Autodesk Fusion 360 part; units mm, degrees
(part 19 of 25)
  line L2175 (67.3326, 33.4819) -> (67.1928, 33.6743)
  arc A5897 (67.71, 32.8087) -> (67.3925, 32.8087) centre (67.5513, 32.8087) ccw
  line L2176 (64.5, 34.1863) -> (63.8511, 34.4551)
  line L2177 (67.5513, 32.8087) -> (67.5141, 33.0437)
  line L2178 (66.1589, 34.2011) -> (66.04, 34.2011)
  line L2179 (59.1947, 30.4591) -> (59.4635, 29.8102)
  line L2180 (67.5513, 30.6913) -> (67.5513, 31.75)
  arc A5898 (59.8478, 29.2014) -> (60.0723, 29.4259) centre (59.9601, 29.3137) ccw
  line L2181 (63.1489, 34.4551) -> (62.5, 34.1863)
  arc A5899 (67.3212, 33.7677) -> (67.0643, 33.581) centre (67.1928, 33.6743) ccw
  arc A5900 (60.0208, 29.4603) -> (59.8993, 29.167) centre (59.9601, 29.3137) ccw
  line L2182 (59.96, 29.3137) -> (60.6089, 29.0449)
  arc A5901 (62.1177, 33.8041) -> (62.3423, 34.0286) centre (62.23, 33.9163) ccw
  arc A5902 (63.2096, 34.3084) -> (63.0881, 34.6018) centre (63.1489, 34.4551) ccw
  arc A5903 (61.8992, 34.0397) -> (62.0207, 34.333) centre (61.9599, 34.1864) ccw
  line L2183 (63.8511, 34.4551) -> (63.1489, 34.4551)
  arc A5904 (65.9211, 34.3598) -> (65.9211, 34.0423) centre (65.9211, 34.2011) ccw
  arc A5905 (64.8373, 33.6244) -> (65.0619, 33.849) centre (64.9496, 33.7367) ccw
  arc A5906 (65.3412, 33.8539) -> (65.1546, 34.1108) centre (65.2479, 33.9824) ccw
  arc A5907 (61.3719, 34.6018) -> (61.2504, 34.3084) centre (61.3112, 34.4551) ccw
  arc A5908 (62.1177, 34.0286) -> (62.3423, 33.8041) centre (62.23, 33.9164) ccw
  arc A5909 (59.3414, 30.5198) -> (59.048, 30.3983) centre (59.1947, 30.4591) ccw
  arc A5910 (66.04, 34.0423) -> (66.04, 34.3598) centre (66.04, 34.2011) ccw
  arc A5911 (62.0722, 34.2986) -> (61.8477, 34.0741) centre (61.9599, 34.1864) ccw
  arc A5912 (62.4393, 34.333) -> (62.5608, 34.0397) centre (62.5001, 34.1864) ccw
  line L2184 (59.1947, 33.0409) -> (59.1947, 30.4591)
  line L2185 (59.96, 34.1863) -> (59.4635, 33.6898)
  line L2186 (65.0555, 33.8426) -> (64.9496, 33.7367)
  line L2187 (65.9211, 34.2011) -> (65.6861, 34.1639)
  arc A5913 (63.8511, 34.2963) -> (63.8511, 34.6138) centre (63.8511, 34.455) ccw
  arc A5914 (65.7352, 34.0129) -> (65.637, 34.3149) centre (65.6861, 34.1639) ccw
  arc A5915 (63.1489, 34.6138) -> (63.1489, 34.2963) centre (63.1489, 34.455) ccw
  line L2188 (59.4635, 33.6898) -> (59.1947, 33.0409)
  arc A5916 (64.8373, 33.849) -> (65.0619, 33.6244) centre (64.9496, 33.7367) ccw
  arc A5917 (65.1758, 34.1238) -> (65.32, 33.8409) centre (65.2479, 33.9824) ccw
  arc A5918 (59.6101, 33.629) -> (59.3168, 33.7505) centre (59.4635, 33.6897) ccw
  arc A5919 (60.5481, 28.8982) -> (60.6696, 29.1916) centre (60.6089, 29.0449) ccw
  arc A5920 (60.6696, 34.3084) -> (60.5481, 34.6018) centre (60.6089, 34.4551) ccw
  arc A5921 (65.4108, 34.2414) -> (65.5089, 33.9394) centre (65.4599, 34.0904) ccw
  arc A5922 (60.0723, 34.0741) -> (59.8478, 34.2986) centre (59.9601, 34.1864) ccw
  line L2189 (65.4599, 34.0904) -> (65.2479, 33.9824)
  arc A5923 (59.3168, 29.7495) -> (59.6101, 29.871) centre (59.4635, 29.8102) ccw
  line L2190 (60.6089, 34.4551) -> (59.96, 34.1863)
  arc A5924 (59.3535, 33.0409) -> (59.036, 33.0409) centre (59.1947, 33.0409) ccw
  arc A5925 (61.3111, 28.8862) -> (61.3111, 29.2037) centre (61.3111, 29.045) ccw
  arc A5926 (62.6123, 34.0741) -> (62.3878, 34.2986) centre (62.5001, 34.1863) ccw
  line L2191 (59.4635, 29.8102) -> (59.96, 29.3137)
  arc A5927 (60.6089, 34.6138) -> (60.6089, 34.2963) centre (60.6089, 34.455) ccw
  arc A5928 (59.5757, 29.9225) -> (59.3512, 29.698) centre (59.4635, 29.8102) ccw
  arc A5929 (64.9621, 33.971) -> (65.1488, 33.7141) centre (65.0555, 33.8426) ccw
  line L2192 (65.6861, 34.1639) -> (65.4599, 34.0904)
  arc A5930 (61.3111, 34.2963) -> (61.3111, 34.6138) centre (61.3111, 34.455) ccw
  line L2193 (62.5, 34.1863) -> (62.23, 33.9163)
  line L2194 (61.3111, 34.4551) -> (60.6089, 34.4551)
  line L2195 (61.96, 34.1863) -> (61.3111, 34.4551)
  arc A5931 (65.5319, 33.9489) -> (65.3878, 34.2318) centre (65.4599, 34.0904) ccw
  arc A5932 (63.9119, 34.6018) -> (63.7904, 34.3084) centre (63.8512, 34.4551) ccw
  line L2196 (62.23, 33.9163) -> (61.96, 34.1863)
  line L2197 (65.2479, 33.9824) -> (65.0555, 33.8426)
  arc A5933 (59.3512, 33.802) -> (59.5757, 33.5775) centre (59.4635, 33.6898) ccw
  arc A5934 (65.1677, 33.7303) -> (64.9432, 33.9548) centre (65.0555, 33.8425) ccw
  arc A5935 (68.4212, 25.4) -> (68.7387, 25.4) centre (68.5799, 25.4) ccw
  line L2198 (67.3481, 25.4) -> (67.3481, 24.8897)
  arc A5936 (62.6433, 28.6748) -> (62.4188, 28.4503) centre (62.5311, 28.5626) ccw
  arc A5937 (69.342, 26.6382) -> (69.342, 26.9558) centre (69.342, 26.797) ccw
  line L2199 (68.58, 25.4) -> (67.3481, 25.4)
  arc A5938 (68.58, 25.5588) -> (68.58, 25.2413) centre (68.58, 25.4001) ccw
  line L2200 (68.58, 26.6319) -> (68.58, 25.4)
  arc A5939 (67.2358, 26.0225) -> (67.4604, 25.798) centre (67.3481, 25.9103) ccw
  line L2201 (67.3481, 25.4) -> (68.58, 25.4)
  arc A5940 (67.1894, 24.8897) -> (67.5069, 24.8897) centre (67.3482, 24.8897) ccw
  arc A5941 (61.2504, 29.1916) -> (61.3719, 28.8982) centre (61.3112, 29.0449) ccw
  arc A5942 (64.4819, 26.6503) -> (64.6034, 26.9437) centre (64.5426, 26.797) ccw
  arc A5943 (61.8477, 29.4259) -> (62.0722, 29.2014) centre (61.9599, 29.3137) ccw
  line L2202 (64.1225, 26.971) -> (64.5426, 26.797)
  arc A5944 (68.4213, 25.4) -> (68.7388, 25.4) centre (68.58, 25.4) ccw
  arc A5945 (62.2447, 29.3444) -> (62.4693, 29.5689) centre (62.357, 29.4567) ccw
  arc A5946 (62.3843, 28.5018) -> (62.6777, 28.6233) centre (62.531, 28.5626) ccw
  line L2203 (62.531, 28.5625) -> (63.801, 27.2925)
  arc A5947 (69.1833, 26.3802) -> (69.5007, 26.3802) centre (69.342, 26.3802) ccw
  line L2204 (64.5426, 26.797) -> (69.342, 26.797)
  arc A5948 (62.1983, 28.9826) -> (62.5158, 28.9826) centre (62.3571, 28.9826) ccw
  arc A5949 (68.58, 26.7906) -> (68.58, 26.4731) centre (68.58, 26.6319) ccw
  arc A5950 (63.9133, 27.4048) -> (63.6888, 27.1803) centre (63.801, 27.2926) ccw
  arc A5951 (67.5069, 25.9103) -> (67.1894, 25.9103) centre (67.3482, 25.9103) ccw
  arc A5952 (62.3423, 29.4714) -> (62.1177, 29.6959) centre (62.23, 29.5836) ccw
  arc A5953 (62.5158, 29.4567) -> (62.1983, 29.4567) centre (62.3571, 29.4567) ccw
  arc A5954 (69.0903, 26.4731) -> (69.0903, 26.7906) centre (69.0903, 26.6319) ccw
  arc A5955 (59.036, 30.4591) -> (59.3535, 30.4591) centre (59.1947, 30.4591) ccw
  arc A5956 (69.5007, 26.797) -> (69.1833, 26.797) centre (69.342, 26.797) ccw
  line L2205 (63.801, 27.2925) -> (64.1225, 26.971)
  arc A5957 (62.0207, 29.167) -> (61.8992, 29.4603) centre (61.9599, 29.3137) ccw
  line L2206 (62.357, 28.9826) -> (62.531, 28.5625)
  arc A5958 (68.4212, 25.4) -> (68.7387, 25.4) centre (68.5799, 25.4) ccw
  line L2207 (68.58, 26.6319) -> (68.0697, 26.6319)
  arc A5959 (64.0103, 26.8588) -> (64.2348, 27.0833) centre (64.1226, 26.9711) ccw
  arc A5960 (68.7387, 25.4) -> (68.4212, 25.4) centre (68.5799, 25.4) ccw
  line L2208 (64.9496, 33.7367) -> (64.5, 34.1863)
  arc A5961 (68.0697, 26.7906) -> (68.0697, 26.4731) centre (68.0697, 26.6319) ccw
  arc A5962 (64.6122, 34.2986) -> (64.3877, 34.0741) centre (64.5, 34.1864) ccw
  arc A5963 (67.3481, 25.5588) -> (67.3481, 25.2413) centre (67.3481, 25.4001) ccw
  line L2209 (62.23, 29.5837) -> (62.357, 29.4567)
  arc A5964 (68.58, 25.2413) -> (68.58, 25.5588) centre (68.58, 25.4001) ccw
  arc A5965 (67.3481, 25.5587) -> (67.3481, 25.2412) centre (67.3481, 25.4) ccw
  arc A5966 (68.58, 25.2413) -> (68.58, 25.5588) centre (68.58, 25.4001) ccw
  line L2210 (69.342, 26.797) -> (69.342, 26.3802)
  arc A5967 (68.58, 25.2412) -> (68.58, 25.5587) centre (68.58, 25.4) ccw
  arc A5968 (68.7387, 26.6319) -> (68.4212, 26.6319) centre (68.5799, 26.6319) ccw
  arc A5969 (62.5037, 29.0434) -> (62.2103, 28.9219) centre (62.357, 28.9827) ccw
  line L2211 (62.357, 29.4567) -> (62.357, 28.9826)
  arc A5970 (69.2297, 26.2679) -> (69.4543, 26.4924) centre (69.342, 26.3801) ccw
  arc A5971 (68.0697, 24.3268) -> (68.0697, 24.0094) centre (68.0697, 24.1681) ccw
  arc A5972 (68.58, 26.4731) -> (68.58, 26.7906) centre (68.58, 26.6319) ccw
  line L2212 (67.437, 18.8226) -> (67.611, 18.4025)
  arc A5973 (68.0768, 21.6936) -> (67.8523, 21.9182) centre (67.9646, 21.8059) ccw
  line L2213 (67.611, 18.4025) -> (67.9325, 18.081)
  line L2214 (68.58, 24.1681) -> (68.58, 25.4)
  arc A5974 (68.182, 26.5196) -> (67.9575, 26.7442) centre (68.0697, 26.6319) ccw
  arc A5975 (68.58, 25.2412) -> (68.58, 25.5587) centre (68.58, 25.4) ccw
  line L2215 (69.0903, 26.6319) -> (68.58, 26.6319)
  line L2216 (68.58, 25.4) -> (68.58, 26.6319)
  line L2217 (69.342, 26.3802) -> (69.0903, 26.6319)
  arc A5976 (72.9775, 15.7587) -> (72.753, 15.5341) centre (72.8653, 15.6464) ccw
  line L2218 (68.58, 25.4) -> (68.58, 24.1681)
  line L2219 (67.0941, 20.9355) -> (67.0941, 19.7045)
  arc A5977 (67.7233, 18.5148) -> (67.4988, 18.2903) centre (67.6111, 18.4026) ccw
  arc A5978 (69.4543, 22.5862) -> (69.2297, 22.8107) centre (69.342, 22.6985) ccw
  arc A5979 (64.5426, 26.9558) -> (64.5426, 26.6382) centre (64.5426, 26.797) ccw
  arc A5980 (68.7387, 25.4) -> (68.4212, 25.4) centre (68.5799, 25.4) ccw
  arc A5981 (70.2539, 15.9671) -> (70.1324, 15.6737) centre (70.1932, 15.8204) ccw
  line L2220 (72.8653, 15.6464) -> (73.2188, 15.2929)
  arc A5982 (69.2025, 26.7441) -> (68.978, 26.5196) centre (69.0902, 26.6319) ccw
  line L2221 (67.3481, 25.9103) -> (67.3481, 25.4)
  line L2222 (73.8677, 15.0241) -> (74.5699, 15.0241)
  arc A5983 (67.1894, 25.4) -> (67.5069, 25.4) centre (67.3482, 25.4) ccw
  line L2223 (73.2188, 15.2929) -> (73.8677, 15.0241)
  arc A5984 (68.58, 25.5587) -> (68.58, 25.2412) centre (68.58, 25.4) ccw
  arc A5985 (60.6089, 29.2037) -> (60.6089, 28.8862) centre (60.6089, 29.045) ccw
  arc A5986 (68.4495, 21.6471) -> (68.4495, 21.9646) centre (68.4495, 21.8059) ccw
  arc A5987 (67.5957, 19.3616) -> (67.2782, 19.3616) centre (67.4369, 19.3616) ccw
  line L2224 (70.6132, 15.6464) -> (72.8653, 15.6464)
  line L2225 (61.96, 29.3137) -> (62.23, 29.5837)
  arc A5988 (64.1833, 27.1177) -> (64.0618, 26.8243) centre (64.1226, 26.971) ccw
  arc A5989 (68.7388, 26.6319) -> (68.4213, 26.6319) centre (68.58, 26.6319) ccw
  arc A5990 (62.3423, 29.6959) -> (62.1177, 29.4714) centre (62.23, 29.5836) ccw
  arc A5991 (63.6888, 27.1803) -> (63.9133, 27.4048) centre (63.801, 27.2926) ccw
  arc A5992 (73.8069, 14.8774) -> (73.9284, 15.1708) centre (73.8676, 15.0241) ccw
  line L2226 (67.0941, 19.7045) -> (67.437, 19.3616)
  arc A5993 (70.0809, 15.7082) -> (70.3054, 15.9327) centre (70.1932, 15.8205) ccw
  line L2227 (61.3111, 29.0449) -> (61.96, 29.3137)
  line L2228 (68.0697, 26.6319) -> (67.3481, 25.9103)
  line L2229 (69.342, 22.6984) -> (68.4495, 21.8059)
  arc A5994 (73.2796, 15.4395) -> (73.1581, 15.1462) centre (73.2189, 15.2929) ccw
  arc A5995 (67.2528, 20.9355) -> (66.9353, 20.9355) centre (67.094, 20.9355) ccw
  arc A5996 (67.9575, 24.0558) -> (68.182, 24.2804) centre (68.0697, 24.1681) ccw
  line L2230 (70.1931, 15.8204) -> (70.6132, 15.6464)
  arc A5997 (69.4543, 24.3076) -> (69.2297, 24.5321) centre (69.342, 24.4199) ccw
  arc A5998 (67.9645, 21.9646) -> (67.9645, 21.6471) centre (67.9645, 21.8059) ccw
  line L2231 (67.9325, 18.081) -> (70.1931, 15.8204)
  arc A5999 (68.3372, 21.9181) -> (68.5617, 21.6936) centre (68.4494, 21.8059) ccw
  arc A6000 (68.0448, 18.1933) -> (67.8203, 17.9688) centre (67.9326, 18.0811) ccw
  arc A6001 (66.9353, 19.7045) -> (67.2528, 19.7045) centre (67.094, 19.7045) ccw
  arc A6002 (72.8653, 15.4877) -> (72.8653, 15.8051) centre (72.8653, 15.6464) ccw
  line L2232 (67.9645, 21.8059) -> (67.0941, 20.9355)
  arc A6003 (68.7388, 25.4) -> (68.4213, 25.4) centre (68.58, 25.4) ccw
  arc A6004 (67.8203, 17.9688) -> (68.0448, 18.1933) centre (67.9326, 18.0811) ccw
  arc A6005 (68.4212, 24.1681) -> (68.7387, 24.1681) centre (68.5799, 24.1681) ccw
  line L2233 (68.0697, 24.1681) -> (68.58, 24.1681)
  arc A6006 (70.6132, 15.8051) -> (70.6132, 15.4877) centre (70.6132, 15.6464) ccw
  arc A6007 (75.6846, 15.5341) -> (75.4601, 15.7587) centre (75.5724, 15.6464) ccw
  arc A6008 (73.5901, 12.446) -> (73.9076, 12.446) centre (73.7489, 12.446) ccw
  arc A6009 (67.2064, 19.8168) -> (66.9818, 19.5923) centre (67.0941, 19.7046) ccw
  arc A6010 (75.2795, 15.1462) -> (75.158, 15.4395) centre (75.2188, 15.2929) ccw
  arc A6011 (67.4643, 18.3418) -> (67.7577, 18.4633) centre (67.611, 18.4025) ccw
  arc A6012 (67.2782, 18.8226) -> (67.5957, 18.8226) centre (67.4369, 18.8226) ccw
  arc A6013 (66.9818, 21.0477) -> (67.2064, 20.8232) centre (67.0941, 20.9354) ccw
  line L2234 (67.437, 19.3616) -> (67.437, 18.8226)
  arc A6014 (69.5007, 24.4198) -> (69.1833, 24.4198) centre (69.342, 24.4198) ccw
  line L2235 (69.342, 24.4198) -> (69.342, 22.6984)
  arc A6015 (73.1066, 15.1806) -> (73.3311, 15.4051) centre (73.2189, 15.2929) ccw
  arc A6016 (72.517, 12.6048) -> (72.517, 12.2873) centre (72.517, 12.4461) ccw
  arc A6017 (68.58, 24.3269) -> (68.58, 24.0094) centre (68.58, 24.1682) ccw
  line L2236 (73.7489, 12.446) -> (73.7489, 12.9563)
  arc A6018 (67.3247, 19.2494) -> (67.5493, 19.4739) centre (67.437, 19.3617) ccw
  line L2237 (72.517, 11.2141) -> (72.517, 12.446)
  arc A6019 (70.5525, 15.4997) -> (70.674, 15.7931) centre (70.6132, 15.6464) ccw
  arc A6020 (69.0903, 24.0094) -> (69.0903, 24.3269) centre (69.0903, 24.1682) ccw
  line L2238 (68.58, 24.1681) -> (69.0903, 24.1681)
  arc A6021 (67.5069, 25.4) -> (67.1894, 25.4) centre (67.3482, 25.4) ccw
  arc A6022 (68.978, 24.2804) -> (69.2025, 24.0558) centre (69.0903, 24.1681) ccw
  line L2239 (69.0903, 24.1681) -> (69.342, 24.4198)
  arc A6023 (69.1833, 22.6984) -> (69.5007, 22.6984) centre (69.342, 22.6984) ccw
  arc A6024 (68.58, 24.0093) -> (68.58, 24.3268) centre (68.58, 24.1681) ccw
  line L2240 (68.4495, 21.8059) -> (67.9645, 21.8059)
  arc A6025 (68.4213, 24.1681) -> (68.7388, 24.1681) centre (68.58, 24.1681) ccw
  arc A6026 (67.4604, 25.002) -> (67.2358, 24.7775) centre (67.3481, 24.8897) ccw
  line L2241 (67.3481, 24.8897) -> (68.0697, 24.1681)
  arc A6027 (67.5837, 18.8834) -> (67.2903, 18.7619) centre (67.437, 18.8226) ccw
  line L2242 (72.517, 13.6779) -> (72.517, 12.446)
  arc A6028 (74.5092, 15.1708) -> (74.6307, 14.8774) centre (74.57, 15.0241) ccw
  arc A6029 (72.6757, 12.446) -> (72.3582, 12.446) centre (72.517, 12.446) ccw
  line L2243 (78.673, 15.2859) -> (74.5249, 11.1379)
  arc A6030 (73.5901, 11.9357) -> (73.9076, 11.9357) centre (73.7489, 11.9357) ccw
  arc A6031 (75.5723, 15.8051) -> (75.5723, 15.4877) centre (75.5723, 15.6464) ccw
  arc A6032 (72.3583, 11.2141) -> (72.6758, 11.2141) centre (72.517, 11.2141) ccw
  arc A6033 (72.517, 11.3728) -> (72.517, 11.0554) centre (72.517, 11.2141) ccw
  line L2244 (74.5249, 11.1379) -> (72.1601, 11.1379)
  line L2245 (73.7489, 12.9563) -> (73.0273, 13.6779)
  line L2246 (75.2188, 15.2929) -> (75.5723, 15.6464)
  arc A6034 (72.517, 13.8366) -> (72.517, 13.5191) centre (72.517, 13.6779) ccw
  arc A6035 (73.7489, 12.2872) -> (73.7489, 12.6047) centre (73.7489, 12.446) ccw
  arc A6036 (72.517, 11.0553) -> (72.517, 11.3728) centre (72.517, 11.2141) ccw
  arc A6037 (73.9076, 12.9563) -> (73.5901, 12.9563) centre (73.7489, 12.9563) ccw
  line L2247 (72.517, 12.446) -> (72.517, 11.2141)
  arc A6038 (78.5607, 15.3982) -> (78.7852, 15.1737) centre (78.673, 15.286) ccw
  arc A6039 (72.1961, 11.3264) -> (71.9716, 11.1018) centre (72.0838, 11.2141) ccw
  line L2248 (73.0273, 13.6779) -> (72.517, 13.6779)
  arc A6040 (79.2149, 15.4997) -> (79.0934, 15.7931) centre (79.1542, 15.6464) ccw
  arc A6041 (73.8612, 11.8235) -> (73.6366, 12.048) centre (73.7489, 11.9358) ccw
  arc A6042 (72.1601, 11.2966) -> (72.1601, 10.9791) centre (72.1601, 11.1379) ccw
  line L2249 (75.5723, 15.6464) -> (79.1542, 15.6464)
  line L2250 (79.1542, 15.6464) -> (78.9481, 15.561)
  arc A6043 (75.1065, 15.4051) -> (75.331, 15.1806) centre (75.2188, 15.2929) ccw
  arc A6044 (79.1542, 15.4877) -> (79.1542, 15.8051) centre (79.1542, 15.6464) ccw
  line L2251 (78.9481, 15.561) -> (78.673, 15.2859)
  arc A6045 (74.5699, 14.8654) -> (74.5699, 15.1829) centre (74.5699, 15.0242) ccw
  arc A6046 (72.3583, 12.446) -> (72.6758, 12.446) centre (72.517, 12.446) ccw
  line L2252 (72.517, 11.2141) -> (73.0273, 11.2141)
  arc A6047 (73.1395, 13.7902) -> (72.915, 13.5656) centre (73.0272, 13.6779) ccw
  arc A6048 (74.5249, 10.9791) -> (74.5249, 11.2966) centre (74.5249, 11.1379) ccw
  arc A6049 (73.8677, 15.1829) -> (73.8677, 14.8654) centre (73.8677, 15.0242) ccw
  arc A6050 (73.9076, 12.446) -> (73.5901, 12.446) centre (73.7489, 12.446) ccw
  arc A6051 (78.8873, 15.7077) -> (79.0088, 15.4144) centre (78.948, 15.5611) ccw
  line L2253 (72.0839, 11.2141) -> (72.517, 11.2141)
  arc A6052 (72.0478, 11.0256) -> (72.2723, 11.2502) centre (72.16, 11.1379) ccw
  arc A6053 (72.517, 12.2872) -> (72.517, 12.6047) centre (72.517, 12.446) ccw
  arc A6054 (74.4127, 11.2502) -> (74.6372, 11.0256) centre (74.525, 11.1379) ccw
  arc A6055 (73.0273, 13.5191) -> (73.0273, 13.8366) centre (73.0273, 13.6779) ccw
  arc A6056 (72.6758, 12.446) -> (72.3583, 12.446) centre (72.517, 12.446) ccw
  arc A6057 (73.6366, 12.844) -> (73.8612, 13.0685) centre (73.7489, 12.9562) ccw
  arc A6058 (72.3582, 11.2141) -> (72.6757, 11.2141) centre (72.517, 11.2141) ccw
  arc A6059 (72.517, 12.6047) -> (72.517, 12.2872) centre (72.517, 12.446) ccw
  arc A6060 (72.3582, 12.446) -> (72.6757, 12.446) centre (72.517, 12.446) ccw
  arc A6061 (73.0273, 11.0554) -> (73.0273, 11.3728) centre (73.0273, 11.2141) ccw
  arc A6062 (78.7852, 15.1737) -> (78.5607, 15.3982) centre (78.673, 15.2859) ccw
  line L2254 (74.5699, 15.0241) -> (75.2188, 15.2929)
  arc A6063 (79.0603, 15.4488) -> (78.8358, 15.6733) centre (78.9481, 15.561) ccw
  line L2255 (73.7489, 11.9357) -> (73.7489, 12.446)
  line L2256 (72.517, 12.446) -> (73.7489, 12.446)
  arc A6064 (72.6757, 12.446) -> (72.3582, 12.446) centre (72.517, 12.446) ccw
  line L2257 (68.4989, 14.799) -> (68.1395, 14.9479)
  arc A6065 (71.1264, 12.0129) -> (71.4438, 12.0129) centre (71.2851, 12.0129) ccw
  arc A6066 (46.6957, 21.6967) -> (46.4024, 21.5752) centre (46.5491, 21.636) ccw
  line L2258 (72.517, 12.446) -> (72.517, 13.6779)
  arc A6067 (46.8566, 21.2765) -> (46.5391, 21.2765) centre (46.6979, 21.2765) ccw
  arc A6068 (72.517, 12.6048) -> (72.517, 12.2873) centre (72.517, 12.4461) ccw
  line L2259 (68.774, 14.5239) -> (68.4989, 14.799)
  arc A6069 (72.517, 12.6047) -> (72.517, 12.2872) centre (72.517, 12.446) ccw
  arc A6070 (68.6153, 14.5239) -> (68.9328, 14.5239) centre (68.7741, 14.5239) ccw
  arc A6071 (68.6618, 14.4117) -> (68.8863, 14.6362) centre (68.774, 14.524) ccw
  arc A6072 (72.915, 11.3264) -> (73.1395, 11.1018) centre (73.0272, 11.2141) ccw
  arc A6073 (46.8102, 18.2973) -> (46.5856, 18.0728) centre (46.6979, 18.185) ccw
  arc A6074 (46.5512, 21.2158) -> (46.8446, 21.3373) centre (46.6979, 21.2765) ccw
  line L2260 (46.6979, 21.2765) -> (46.549, 21.6359)
  line L2261 (72.0067, 13.6779) -> (71.2851, 12.9563)
  line L2262 (73.0273, 11.2141) -> (73.7489, 11.9357)
  arc A6075 (49.9351, 15.1066) -> (49.9351, 14.7891) centre (49.9351, 14.9479) ccw
  arc A6076 (68.8863, 14.6362) -> (68.6618, 14.4117) centre (68.7741, 14.5239) ccw
  arc A6077 (68.4382, 14.6524) -> (68.5597, 14.9457) centre (68.499, 14.7991) ccw
  line L2263 (49.9351, 14.9479) -> (46.6979, 18.1851)
  arc A6078 (72.3583, 12.446) -> (72.6758, 12.446) centre (72.517, 12.446) ccw
  arc A6079 (72.6757, 13.6779) -> (72.3582, 13.6779) centre (72.517, 13.6779) ccw
  arc A6080 (73.7489, 12.2873) -> (73.7489, 12.6048) centre (73.7489, 12.4461) ccw
  line L2264 (71.2851, 12.9563) -> (71.2851, 12.446)
  line L2265 (71.2851, 12.0129) -> (68.774, 14.5239)
  arc A6081 (72.6758, 12.446) -> (72.3583, 12.446) centre (72.517, 12.446) ccw
  line L2266 (73.7489, 12.446) -> (72.517, 12.446)
  line L2267 (72.1601, 11.1379) -> (72.0839, 11.2141)
  arc A6082 (72.0839, 11.3728) -> (72.0839, 11.0554) centre (72.0839, 11.2141) ccw
  arc A6083 (46.5391, 18.1851) -> (46.8566, 18.1851) centre (46.6979, 18.1851) ccw
  arc A6084 (72.517, 12.2873) -> (72.517, 12.6048) centre (72.517, 12.4461) ccw
  line L2268 (46.6979, 18.1851) -> (46.6979, 21.2765)
  arc A6085 (71.1728, 11.9006) -> (71.3974, 12.1251) centre (71.2851, 12.0129) ccw
  line L2269 (71.2851, 12.446) -> (71.2851, 12.0129)
  arc A6086 (72.3582, 12.446) -> (72.6757, 12.446) centre (72.517, 12.446) ccw
  arc A6087 (37.5797, 23.0188) -> (37.5797, 22.7012) centre (37.5797, 22.86) ccw
  arc A6088 (72.517, 13.5191) -> (72.517, 13.8366) centre (72.517, 13.6779) ccw
  arc A6089 (44.69, 23.6538) -> (44.69, 23.3362) centre (44.69, 23.495) ccw
  arc A6090 (36.0803, 22.7012) -> (36.0803, 23.0188) centre (36.0803, 22.86) ccw
  arc A6091 (29.21, 23.6538) -> (29.21, 23.3362) centre (29.21, 23.495) ccw
  arc A6092 (71.2851, 12.6047) -> (71.2851, 12.2872) centre (71.2851, 12.446) ccw
  arc A6093 (56.8579, 23.0188) -> (56.8579, 22.7012) centre (56.8579, 22.86) ccw
  line L2270 (71.2851, 12.446) -> (72.517, 12.446)
  arc A6094 (68.6112, 14.9113) -> (68.3867, 14.6868) centre (68.499, 14.799) ccw
  arc A6095 (72.517, 12.2872) -> (72.517, 12.6047) centre (72.517, 12.446) ccw
  arc A6096 (41.924, 23.3362) -> (41.924, 23.6538) centre (41.924, 23.495) ccw
  arc A6097 (49.8228, 14.8356) -> (50.0473, 15.0602) centre (49.9351, 14.9479) ccw
  arc A6098 (71.4438, 12.9563) -> (71.1264, 12.9563) centre (71.2851, 12.9563) ccw
  arc A6099 (32.4997, 23.0188) -> (32.4997, 22.7012) centre (32.4997, 22.86) ccw
  arc A6100 (47.5103, 22.7012) -> (47.5103, 23.0188) centre (47.5103, 22.86) ccw
  arc A6101 (68.2003, 15.0946) -> (68.0788, 14.8012) centre (68.1395, 14.9479) ccw
  arc A6102 (25.1591, 23.3362) -> (25.1591, 23.6538) centre (25.1591, 23.495) ccw
  arc A6103 (38.3409, 23.6538) -> (38.3409, 23.3362) centre (38.3409, 23.495) ccw
  arc A6104 (46.7491, 23.3362) -> (46.7491, 23.6538) centre (46.7491, 23.495) ccw
  line L2271 (72.517, 13.6779) -> (72.0067, 13.6779)
  arc A6105 (72.6758, 13.6779) -> (72.3583, 13.6779) centre (72.517, 13.6779) ccw
  arc A6106 (49.0097, 23.0188) -> (49.0097, 22.7012) centre (49.0097, 22.86) ccw
  line L2272 (72.517, 12.446) -> (71.2851, 12.446)
  arc A6107 (6.2857, 22.7012) -> (6.2857, 23.0188) centre (6.2857, 22.86) ccw
  arc A6108 (69.342, 22.7012) -> (69.342, 23.0188) centre (69.342, 22.86) ccw
  arc A6109 (68.1395, 14.7891) -> (68.1395, 15.1066) centre (68.1395, 14.9479) ccw
  arc A6110 (29.21, 23.3362) -> (29.21, 23.6538) centre (29.21, 23.495) ccw
  arc A6111 (72.0067, 13.8366) -> (72.0067, 13.5191) centre (72.0067, 13.6779) ccw
  arc A6112 (72.119, 13.5656) -> (71.8945, 13.7902) centre (72.0068, 13.6779) ccw
  arc A6113 (71.1264, 12.446) -> (71.4438, 12.446) centre (71.2851, 12.446) ccw
  arc A6114 (71.1728, 13.0685) -> (71.3974, 12.844) centre (71.2851, 12.9563) ccw
  arc A6115 (71.4438, 12.446) -> (71.1264, 12.446) centre (71.2851, 12.446) ccw
  arc A6116 (71.2851, 12.6048) -> (71.2851, 12.2873) centre (71.2851, 12.4461) ccw
  line L2273 (46.549, 21.6359) -> (46.2739, 21.911)
  line L2274 (12.3063, 33.5781) -> (12.5596, 32.9666)
  line L2275 (68.1395, 14.9479) -> (49.9351, 14.9479)
  arc A6117 (72.517, 12.2873) -> (72.517, 12.6048) centre (72.517, 12.4461) ccw
  arc A6118 (0.7747, 23.6538) -> (0.7747, 23.3362) centre (0.7747, 23.495) ccw
  arc A6119 (68.9328, 14.5239) -> (68.6153, 14.5239) centre (68.7741, 14.5239) ccw
  arc A6120 (7.62, 23.0188) -> (7.62, 22.7012) centre (7.62, 22.86) ccw
  arc A6121 (79.8488, 22.7012) -> (79.8488, 23.0188) centre (79.8488, 22.86) ccw
  arc A6122 (71.628, 24.2888) -> (71.628, 23.9713) centre (71.628, 24.1301) ccw
  arc A6123 (54.9021, 23.3362) -> (54.9021, 23.6538) centre (54.9021, 23.495) ccw
  arc A6124 (54.5068, 23.6538) -> (54.5068, 23.3362) centre (54.5068, 23.495) ccw
  arc A6125 (84.2253, 22.7012) -> (84.2253, 23.0188) centre (84.2253, 22.86) ccw
  arc A6126 (53.34, 23.3362) -> (53.34, 23.6538) centre (53.34, 23.495) ccw
  arc A6127 (71.628, 23.0188) -> (71.628, 22.7012) centre (71.628, 22.86) ccw
  arc A6128 (45.325, 23.0188) -> (45.325, 22.7012) centre (45.325, 22.86) ccw
  arc A6129 (25.9203, 22.7012) -> (25.9203, 23.0188) centre (25.9203, 22.86) ccw
  arc A6130 (33.5403, 22.7012) -> (33.5403, 23.0188) centre (33.5403, 22.86) ccw
  arc A6131 (42.559, 22.7012) -> (42.559, 23.0188) centre (42.559, 22.86) ccw
  arc A6132 (75.0912, 23.0188) -> (75.0912, 22.7012) centre (75.0912, 22.86) ccw
  arc A6133 (73.3464, 22.7012) -> (73.3464, 23.0188) centre (73.3464, 22.86) ccw
  arc A6134 (83.5279, 23.0188) -> (83.5279, 22.7012) centre (83.5279, 22.86) ccw
  arc A6135 (83.298, 22.3838) -> (83.298, 22.0663) centre (83.298, 22.2251) ccw
  arc A6136 (53.34, 23.6538) -> (53.34, 23.3362) centre (53.34, 23.495) ccw
  arc A6137 (0.7747, 23.0188) -> (0.7747, 22.7012) centre (0.7747, 22.86) ccw
  arc A6138 (27.4197, 23.0188) -> (27.4197, 22.7012) centre (27.4197, 22.86) ccw
  arc A6139 (54.9021, 22.7012) -> (54.9021, 23.0188) centre (54.9021, 22.86) ccw
  arc A6140 (7.62, 22.7012) -> (7.62, 23.0188) centre (7.62, 22.86) ccw
  arc A6141 (71.628, 22.3838) -> (71.628, 22.0663) centre (71.628, 22.2251) ccw
  arc A6142 (8.9543, 23.0188) -> (8.9543, 22.7012) centre (8.9543, 22.86) ccw
  arc A6143 (31.0003, 22.7012) -> (31.0003, 23.0188) centre (31.0003, 22.86) ccw
  arc A6144 (35.0397, 23.0188) -> (35.0397, 22.7012) centre (35.0397, 22.86) ccw
  arc A6145 (51.5497, 23.0188) -> (51.5497, 22.7012) centre (51.5497, 22.86) ccw
  arc A6146 (50.0503, 22.7012) -> (50.0503, 23.0188) centre (50.0503, 22.86) ccw
  arc A6147 (84.2253, 22.0663) -> (84.2253, 22.3838) centre (84.2253, 22.2251) ccw
  arc A6148 (44.972, 24.6062) -> (44.972, 24.9238) centre (44.972, 24.765) ccw
  arc A6149 (81.5721, 23.3362) -> (81.5721, 23.6538) centre (81.5721, 23.495) ccw
  arc A6150 (46.4947, 23.9713) -> (46.4947, 24.2888) centre (46.4947, 24.1301) ccw
  arc A6151 (29.21, 24.9238) -> (29.21, 24.6062) centre (29.21, 24.765) ccw
  arc A6152 (54.9021, 24.6062) -> (54.9021, 24.9238) centre (54.9021, 24.765) ccw
  arc A6153 (59.8864, 24.9238) -> (59.8864, 24.6062) centre (59.8864, 24.765) ccw
  arc A6154 (72.39, 24.6062) -> (72.39, 24.9238) centre (72.39, 24.765) ccw
  arc A6155 (56.8579, 23.6538) -> (56.8579, 23.3362) centre (56.8579, 23.495) ccw
  arc A6156 (24.9047, 23.9713) -> (24.9047, 24.2888) centre (24.9047, 24.1301) ccw
  arc A6157 (56.9536, 24.6062) -> (56.9536, 24.9238) centre (56.9536, 24.765) ccw
  arc A6158 (84.2253, 23.9713) -> (84.2253, 24.2888) centre (84.2253, 24.1301) ccw
  arc A6159 (40.816, 24.6062) -> (40.816, 24.9238) centre (40.816, 24.765) ccw
  arc A6160 (68.58, 24.6062) -> (68.58, 24.9238) centre (68.58, 24.765) ccw
  arc A6161 (53.34, 24.2888) -> (53.34, 23.9713) centre (53.34, 24.1301) ccw
  arc A6162 (44.055, 24.2888) -> (44.055, 23.9713) centre (44.055, 24.1301) ccw
  arc A6163 (43.42, 24.9238) -> (43.42, 24.6062) centre (43.42, 24.765) ccw
  arc A6164 (53.34, 24.9238) -> (53.34, 24.6062) centre (53.34, 24.765) ccw
  arc A6165 (69.342, 23.9713) -> (69.342, 24.2888) centre (69.342, 24.1301) ccw
  arc A6166 (41.289, 23.9713) -> (41.289, 24.2888) centre (41.289, 24.1301) ccw
  arc A6167 (57.5886, 23.9713) -> (57.5886, 24.2888) centre (57.5886, 24.1301) ccw
  arc A6168 (54.9021, 23.9713) -> (54.9021, 24.2888) centre (54.9021, 24.1301) ccw
  arc A6169 (38.5953, 24.9238) -> (38.5953, 24.6062) centre (38.5953, 24.765) ccw
  arc A6170 (54.8513, 24.9238) -> (54.8513, 24.6062) centre (54.8513, 24.765) ccw
  arc A6171 (72.39, 24.9238) -> (72.39, 24.6062) centre (72.39, 24.765) ccw
  arc A6172 (53.34, 24.6062) -> (53.34, 24.9238) centre (53.34, 24.765) ccw
  arc A6173 (67.4728, 24.6062) -> (67.4728, 24.9238) centre (67.4728, 24.765) ccw
  arc A6174 (68.58, 24.9238) -> (68.58, 24.6062) centre (68.58, 24.765) ccw
  arc A6175 (54.8178, 24.2888) -> (54.8178, 23.9713) centre (54.8178, 24.1301) ccw
  arc A6176 (71.628, 23.6538) -> (71.628, 23.3362) centre (71.628, 23.495) ccw
  arc A6177 (0.7747, 24.2888) -> (0.7747, 23.9713) centre (0.7747, 24.1301) ccw
  arc A6178 (83.5279, 24.2888) -> (83.5279, 23.9713) centre (83.5279, 24.1301) ccw
  arc A6179 (54.9021, 25.2413) -> (54.9021, 25.5588) centre (54.9021, 25.4001) ccw
  arc A6180 (59.2514, 24.2888) -> (59.2514, 23.9713) centre (59.2514, 24.1301) ccw
  arc A6181 (83.5279, 23.6538) -> (83.5279, 23.3362) centre (83.5279, 23.495) ccw
  arc A6182 (43.1637, 25.5588) -> (43.1637, 25.2413) centre (43.1637, 25.4001) ccw
  arc A6183 (0.7747, 24.9238) -> (0.7747, 24.6062) centre (0.7747, 24.765) ccw
  arc A6184 (81.5721, 23.9713) -> (81.5721, 24.2888) centre (81.5721, 24.1301) ccw
  arc A6185 (56.8579, 24.2888) -> (56.8579, 23.9713) centre (56.8579, 24.1301) ccw
  arc A6186 (84.0359, 25.5588) -> (84.0359, 25.2413) centre (84.0359, 25.4001) ccw
  arc A6187 (59.8864, 26.1938) -> (59.8864, 25.8762) centre (59.8864, 26.035) ccw
  arc A6188 (29.21, 24.2888) -> (29.21, 23.9713) centre (29.21, 24.1301) ccw
  arc A6189 (84.2253, 23.3362) -> (84.2253, 23.6538) centre (84.2253, 23.495) ccw
  arc A6190 (56.8579, 24.9238) -> (56.8579, 24.6062) centre (56.8579, 24.765) ccw
  arc A6191 (68.58, 25.8762) -> (68.58, 26.1938) centre (68.58, 26.035) ccw
  arc A6192 (15.4854, 24.6062) -> (15.4854, 24.9238) centre (15.4854, 24.765) ccw
  arc A6193 (73.4972, 26.1938) -> (73.4972, 25.8762) centre (73.4972, 26.035) ccw
  arc A6194 (14.7483, 25.8762) -> (14.7483, 26.1938) centre (14.7483, 26.035) ccw
  arc A6195 (68.58, 25.2413) -> (68.58, 25.5588) centre (68.58, 25.4001) ccw
  arc A6196 (84.0164, 26.1938) -> (84.0164, 25.8762) centre (84.0164, 26.035) ccw
  arc A6197 (69.342, 23.3362) -> (69.342, 23.6538) centre (69.342, 23.495) ccw
  arc A6198 (53.34, 23.9713) -> (53.34, 24.2888) centre (53.34, 24.1301) ccw
  arc A6199 (38.5953, 25.5588) -> (38.5953, 25.2413) centre (38.5953, 25.4001) ccw
  arc A6200 (59.9059, 25.5588) -> (59.9059, 25.2413) centre (59.9059, 25.4001) ccw
  arc A6201 (38.5953, 24.2888) -> (38.5953, 23.9713) centre (38.5953, 24.1301) ccw
  arc A6202 (29.21, 24.6062) -> (29.21, 24.9238) centre (29.21, 24.765) ccw
  arc A6203 (43.702, 25.8762) -> (43.702, 26.1938) centre (43.702, 26.035) ccw
  arc A6204 (53.34, 25.8762) -> (53.34, 26.1938) centre (53.34, 26.035) ccw
  arc A6205 (81.0836, 24.6062) -> (81.0836, 24.9238) centre (81.0836, 24.765) ccw
  arc A6206 (53.34, 25.5588) -> (53.34, 25.2413) centre (53.34, 25.4001) ccw
  arc A6207 (14.8554, 25.2413) -> (14.8554, 25.5588) centre (14.8554, 25.4001) ccw
  arc A6208 (72.39, 26.1938) -> (72.39, 25.8762) centre (72.39, 26.035) ccw
  arc A6209 (14.991, 26.5113) -> (14.991, 26.8288) centre (14.991, 26.67) ccw
  arc A6210 (72.39, 25.8762) -> (72.39, 26.1938) centre (72.39, 26.035) ccw
  arc A6211 (29.21, 23.9713) -> (29.21, 24.2888) centre (29.21, 24.1301) ccw
  arc A6212 (40.6563, 25.2413) -> (40.6563, 25.5588) centre (40.6563, 25.4001) ccw
  arc A6213 (54.8513, 26.1938) -> (54.8513, 25.8762) centre (54.8513, 26.035) ccw
  arc A6214 (0.7747, 25.5588) -> (0.7747, 25.2413) centre (0.7747, 25.4001) ccw
  arc A6215 (84.2253, 25.8762) -> (84.2253, 26.1938) centre (84.2253, 26.035) ccw
  arc A6216 (53.34, 26.1938) -> (53.34, 25.8762) centre (53.34, 26.035) ccw
  arc A6217 (68.58, 26.1938) -> (68.58, 25.8762) centre (68.58, 26.035) ccw
  arc A6218 (29.21, 26.1938) -> (29.21, 25.8762) centre (29.21, 26.035) ccw
  arc A6219 (0.7747, 26.1938) -> (0.7747, 25.8762) centre (0.7747, 26.035) ccw
  arc A6220 (44.337, 25.2413) -> (44.337, 25.5588) centre (44.337, 25.4001) ccw
  arc A6221 (56.9536, 25.8762) -> (56.9536, 26.1938) centre (56.9536, 26.035) ccw
  arc A6222 (0.7747, 26.8288) -> (0.7747, 26.5113) centre (0.7747, 26.67) ccw
  arc A6223 (37.5797, 28.0988) -> (37.5797, 27.7813) centre (37.5797, 27.9401) ccw
  arc A6224 (54.9021, 27.7813) -> (54.9021, 28.0988) centre (54.9021, 27.9401) ccw
  arc A6225 (51.943, 28.0988) -> (51.943, 27.7813) centre (51.943, 27.9401) ccw
  arc A6226 (84.2253, 26.5113) -> (84.2253, 26.8288) centre (84.2253, 26.67) ccw
  arc A6227 (83.3814, 26.8288) -> (83.3814, 26.5113) centre (83.3814, 26.67) ccw
  arc A6228 (84.0164, 24.9238) -> (84.0164, 24.6062) centre (84.0164, 24.765) ccw
  arc A6229 (56.8579, 26.1938) -> (56.8579, 25.8762) centre (56.8579, 26.035) ccw
  arc A6230 (40.816, 25.8762) -> (40.816, 26.1938) centre (40.816, 26.035) ccw
  arc A6231 (43.004, 26.1938) -> (43.004, 25.8762) centre (43.004, 26.035) ccw
  arc A6232 (73.4972, 24.9238) -> (73.4972, 24.6062) centre (73.4972, 24.765) ccw
  arc A6233 (56.8579, 25.5588) -> (56.8579, 25.2413) centre (56.8579, 25.4001) ccw
  arc A6234 (38.5953, 26.1938) -> (38.5953, 25.8762) centre (38.5953, 26.035) ccw
  arc A6235 (81.0836, 25.8762) -> (81.0836, 26.1938) centre (81.0836, 26.035) ccw
  arc A6236 (84.2253, 25.2413) -> (84.2253, 25.5588) centre (84.2253, 25.4001) ccw
  arc A6237 (84.2253, 24.6062) -> (84.2253, 24.9238) centre (84.2253, 24.765) ccw
  arc A6238 (54.9021, 25.8762) -> (54.9021, 26.1938) centre (54.9021, 26.035) ccw
  arc A6239 (81.0641, 25.2413) -> (81.0641, 25.5588) centre (81.0641, 25.4001) ccw
  arc A6240 (29.21, 25.8762) -> (29.21, 26.1938) centre (29.21, 26.035) ccw
  arc A6241 (72.39, 25.5588) -> (72.39, 25.2413) centre (72.39, 25.4001) ccw
  arc A6242 (56.9341, 25.2413) -> (56.9341, 25.5588) centre (56.9341, 25.4001) ccw
  arc A6243 (67.4728, 25.8762) -> (67.4728, 26.1938) centre (67.4728, 26.035) ccw
  arc A6244 (29.21, 27.1462) -> (29.21, 27.4638) centre (29.21, 27.305) ccw
  arc A6245 (84.2253, 27.7813) -> (84.2253, 28.0988) centre (84.2253, 27.9401) ccw
  arc A6246 (43.067, 26.5113) -> (43.067, 26.8288) centre (43.067, 26.67) ccw
  arc A6247 (36.0803, 27.7813) -> (36.0803, 28.0988) centre (36.0803, 27.9401) ccw
  arc A6248 (81.7186, 26.5113) -> (81.7186, 26.8288) centre (81.7186, 26.67) ccw
  arc A6249 (53.34, 27.4638) -> (53.34, 27.1462) centre (53.34, 27.305) ccw
  arc A6250 (41.797, 27.7813) -> (41.797, 28.0988) centre (41.797, 27.9401) ccw
  arc A6251 (73.3714, 27.4638) -> (73.3714, 27.1462) centre (73.3714, 27.305) ccw
  arc A6252 (38.5953, 26.8288) -> (38.5953, 26.5113) centre (38.5953, 26.67) ccw
  arc A6253 (63.1536, 27.7813) -> (63.1536, 28.0988) centre (63.1536, 27.9401) ccw
  arc A6254 (27.813, 28.0988) -> (27.813, 27.7813) centre (27.813, 27.9401) ccw
  arc A6255 (42.432, 27.1462) -> (42.432, 27.4638) centre (42.432, 27.305) ccw
  arc A6256 (84.2253, 27.1462) -> (84.2253, 27.4638) centre (84.2253, 27.305) ccw
  arc A6257 (54.9021, 26.5113) -> (54.9021, 26.8288) centre (54.9021, 26.67) ccw
  arc A6258 (57.5886, 26.5113) -> (57.5886, 26.8288) centre (57.5886, 26.67) ccw
  arc A6259 (56.8579, 28.0988) -> (56.8579, 27.7813) centre (56.8579, 27.9401) ccw
  arc A6260 (29.21, 26.5113) -> (29.21, 26.8288) centre (29.21, 26.67) ccw
  arc A6261 (53.34, 26.5113) -> (53.34, 26.8288) centre (53.34, 26.67) ccw
  arc A6262 (5.9265, 27.7813) -> (5.9265, 28.0988) centre (5.9265, 27.9401) ccw
  arc A6263 (69.342, 26.5113) -> (69.342, 26.8288) centre (69.342, 26.67) ccw
  arc A6264 (33.5403, 27.7813) -> (33.5403, 28.0988) centre (33.5403, 27.9401) ccw
  arc A6265 (29.21, 26.8288) -> (29.21, 26.5113) centre (29.21, 26.67) ccw